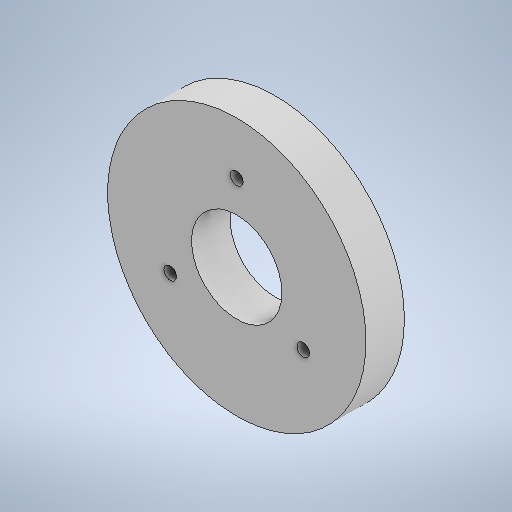
# Autodesk Inventor part: 旋钮帽基座-v0.1.0
Saved by Autodesk Inventor 2025 (Build 290162000, 162)
## iProperties
Created: 2025-05-09
Part Number: 旋钮帽基座-v0.1.0
Material: 常规
Document SubType Name: Modeling
Designer: hawav
Density: 1 g/cm^3
Appearance: 默认
Author: hawav
Autodesk Inventor part; units mm, degrees
ref_plane "YZ Plane" through (0, 0, 0) normal (1, 0, 0) x (0, 1, 0)
ref_plane "XZ Plane" through (0, 0, 0) normal (0, 1, 0) x (-1, 0, 0)
ref_plane "XY Plane" through (0, 0, 0) normal (0, 0, 1) x (1, 0, 0)
sketch "草图1" plane through (0, 0, 0) normal (0, 0, 1) x (1, 0, 0)
  circle A0 centre (0, 0) radius 33.6
  circle A1 centre (0, 0) radius 20
  circle A2 centre (0, 20) radius 1.65
  circle A3 centre (-17.3205, -10) radius 1.65
  circle A4 centre (17.3205, -10) radius 1.65
  circle A5 centre (0, 0) radius 11.75
  dimension "d1" = 40
  dimension "d0" = 67.2
  dimension "d2" = 3.3
  dimension "d5" = 360
  dimension "d7" = 23.5
  constraints: 5 centre point, 3 coincident, 1 vertical alignment, 9 other
  measures "d0" diameter of A0
  measures "d2" diameter of A2
  measures "d7" diameter of A5
extrude "拉伸1" add sketch "草图1" along normal blind 10 contours A0 | A1 A4 A3 A2
